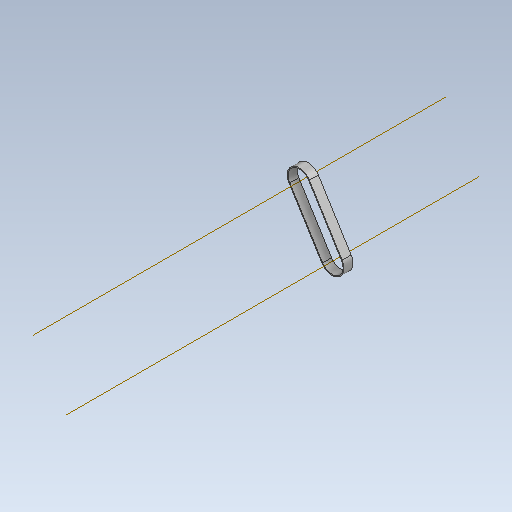
# Autodesk Inventor part: Synchronous Belt
Saved by Autodesk Inventor 2020 (Build 240168000, 168)
## iProperties
Created: 2022-07-22
Part Number: Synchronous Belt
Material: Rubber
Document SubType Name: Modeling
Designer: iPICLab4
Density: 1 g/cm^3
Appearance: Rubber - Black - Version 1.1
CustomPartVersion: 1
Author: iPICLab4
Autodesk Inventor part; units mm, degrees
sketch "Sketch Path" plane through (0, 0, 0) normal (0, 0, 1) x (1, 0, 0)
  arc A0 (37.1866, -44.5957) -> (23.4466, -53.1213) centre (30.3166, -48.8585) ccw
  arc A1 (46.6455, -90.5087) -> (60.3854, -81.983) centre (53.5154, -86.2459) ccw
  line L0 (46.6455, -90.5087) -> (23.4466, -53.1213)
  line L1 (37.1866, -44.5957) -> (60.3854, -81.983)
  constraints: 4 end point, 4 point on circle, 2 centre point
ref_plane "Cross Section Plane" through (23.4466, -53.1213, 0) normal (0.5272, -0.8497, 0) x (0, 0, 1)
ref_plane "Work Plane2" through (30.3166, -48.8585, 0) normal (-1, 0, 0) x (0, 0, 1)
ref_plane "Work Plane3" through (53.5154, -86.2459, 0) normal (-0.4604, 0.8877, 0) x (0, 0, 1)
sketch "Cross Section" plane through (23.4466, -53.1213, 0) normal (0.5272, -0.8497, 0) x (0, 0, 1)
  line L0 (-3.175, 0.381) -> (3.175, 0.381)
  line L1 (3.175, 0.381) -> (3.175, -0.254)
  line L2 (3.175, -0.254) -> (-3.175, -0.254)
  line L3 (-3.175, -0.254) -> (-3.175, 0.381)
  line L4 (-3.175, 0) -> (3.175, 0) construction
  point P0 (0, 0)
  point P1 (0, 0)
  dimension "d0" = 6.35
  dimension "d4" = 0.254
  dimension "d5" = 0.381
  constraints: 10 end point, 2 parallel, 2 point on line, 1 coincident, 1 horizontal, 1 midpoint, 1 perpendicular, 1 other
  measures "d0" distance between parallel lines of L1 L3
  measures "d4" distance between parallel lines of L2 L4
  measures "d5" distance between parallel lines of L4 L0
sweep "Belt" add profiles "Cross Section" path "Sketch Path"
equation "\"d0\" = da_B"
equation "\"d4\" = da_a"
equation "\"d5\" = da_a2"
equation "\"da_B\" = 6.35"
equation "\"da_pb\" = 2.032"
equation "\"da_L\" = 138.8"
equation "\"da_a\" = 0.254"
equation "\"da_S\" = 1.143"
equation "\"da_Beta\" = 20deg"
equation "\"da_Ht\" = 0.508"
equation "\"da_H\" = 1.143"
equation "\"da_a2\" = 0.381"
body "Solid1"
